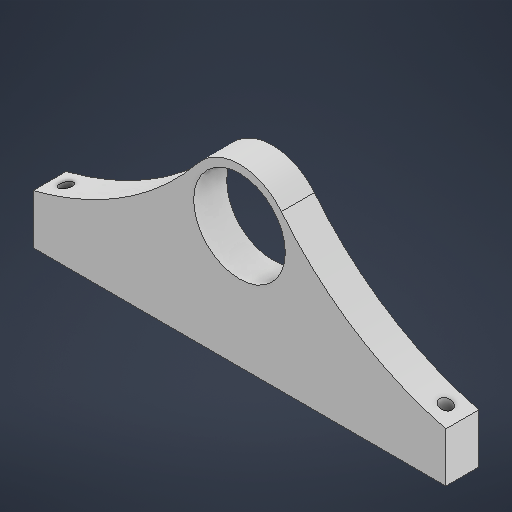
# Autodesk Inventor part: podstawa
Saved by Autodesk Inventor 2026.2 (Build 302298000, 298)
## iProperties
Created: 2025-11-25
Part Number: podstawa
Material: Generic
Document SubType Name: Modeling
Designer: janek
Density: 1 g/cm^3
Appearance: Default
Author: janek
Autodesk Inventor part; units mm, degrees
ref_plane "YZ Plane" through (0, 0, 0) normal (1, 0, 0) x (0, 1, 0)
ref_plane "XZ Plane" through (0, 0, 0) normal (0, 1, 0) x (-1, 0, 0)
ref_plane "XY Plane" through (0, 0, 0) normal (0, 0, 1) x (1, 0, 0)
sketch "Sketch1" plane through (0, 0, 0) normal (0, 0, 1) x (1, 0, 0)
  line L0 (0, 0) -> (100, 0)
  line L1 (100, 0) -> (100, 12)
  line L2 (100, 12) -> (0, 12)
  line L3 (0, 12) -> (0, 0)
  line L4 (37, 12) -> (63, 12)
  line L5 (63, 12) -> (63, 29.5314)
  line L6 (63, 29.5314) -> (37, 29.5314)
  line L7 (37, 29.5314) -> (37, 12)
  circle A0 centre (50, 29.5314) radius 13
  arc A1 (0, 12) -> (39.8482, 37.6517) centre (-18.2502, 84.1269) ccw
  arc A2 (60.1516, 37.652) -> (100, 12) centre (118.2502, 84.1269) ccw
  circle A3 centre (50, 29.5314) radius 11.1
  point P0 (100, 6)
  point P1 (0, 6)
  dimension "d30" = 100
  dimension "d31" = 22.2
  dimension "d32" = 74.4
  dimension "d33" = 74.4
  dimension "d34" = 26
  dimension "d37" = 12
  dimension "d39" = 25.6517
  dimension "d40" = 25.652
  dimension "d41" = 26
  dimension "d43" = 37
  constraints: 16 end point, 7 point on circle, 4 centre point, 4 parallel, 3 midpoint, 2 horizontal, 2 perpendicular, 1 coincident, 1 point on line, 1 tangent
  measures "d30" distance of L1.end L2.end
  measures "d31" diameter of A3
  measures "d32" radius of A2
  measures "d33" radius of A1
  measures "d34" diameter of A0
  measures "d37" distance between parallel lines of L0 L2
  measures "d39" distance from line of L2 A0.end
  measures "d40" distance from line of L2 A2.start
  measures "d41" distance between parallel lines of L5 L7
  measures "d43" distance between parallel lines of L3 L7
extrude "Extrusion1" add sketch "Sketch1" along normal blind 8 contours L3 L2 L1 L0 | A1 A0 L7 L2 | L2 L5 A0 A2 | L7 A0 L5 L2 | A0 L6 A3 | L6 A3 A0
sketch "Sketch2" plane through (0, 0, 0) normal (0, -1, 0) x (1, 0, 0)
  line L0 (0, 8) -> (100, 8) projected
  line L1 (0, 0) -> (0, 8) projected
  line L2 (100, 0) -> (100, 8) projected
  point P0 (4, 4)
  point P1 (96, 4)
  point P2 (100, 4)
  dimension "d12" = 4
  dimension "d13" = 4
  dimension "d14" = 4
  dimension "d15" = 4
  constraints: 1 midpoint
  measures "d12" distance from line of L0 point (4, 4)
  measures "d13" distance from line of L1 point (4, 4)
  measures "d14" distance of point (100, 4) point (96, 4)
  measures "d15" distance from line of L0 point (96, 4)
hole "Hole2" at (4, 0, 4) at (96, 0, 4) direction (0, 1, 0) diameter 3 end through all
body "Solid1"
